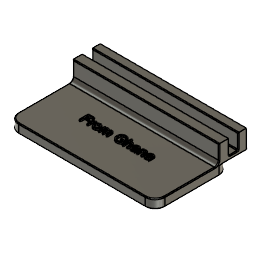
name_tag (Autodesk Fusion 360 design; units mm, degrees)
Autodesk Fusion 360 part; units mm, degrees
sketch "Sketch1" plane through (0, 0, 0) normal (0, 0, 1) x (1, 0, 0)
  line L0 (0, 0) -> (0, 18.796)
  line L1 (0, 0) -> (-86.8649, 0) construction
  line L2 (3.429, 22.225) -> (47.371, 22.225)
  line L3 (25.4, 22.225) -> (25.4, 6.2788) construction
  line L4 (0, 9.398) -> (48.3503, 9.398) construction
  line L5 (3.429, -3.429) -> (47.371, -3.429)
  line L6 (50.8, 0) -> (50.8, 18.796)
  arc A0 (3.429, 22.225) -> (0, 18.796) centre (3.429, 18.796) ccw
  arc A1 (50.8, 18.796) -> (47.371, 22.225) centre (47.371, 18.796) ccw
  arc A2 (47.371, -3.429) -> (50.8, 0) centre (47.371, 0) ccw
  arc A3 (0, 0) -> (3.429, -3.429) centre (3.429, 0) ccw
  dimension "d1" = 18.796
  dimension "d2" = 6.858
  dimension "d3" = 43.942
  constraint coincident L0.start L1.start
  constraint vertical L0
  constraint perpendicular L0 L1
  constraint tangent L0 A0
  constraint horizontal L2
  constraint tangent L2 A0
  constraint midpoint L2 L3.start
  constraint perpendicular L2 L3
  constraint midpoint L0 L4.start
  constraint perpendicular L3 L4
  constraint symmetric L2.start L4 L5.start
  constraint symmetric L2.end L4 L5.end
  constraint symmetric L0.start L3 L6.start
  constraint symmetric L0.end L3 L6.end
  constraint symmetric L3 A0 A1
  constraint symmetric L4 A0 A3
  constraint symmetric L4 A1 A2
  constraint coincident L0 L1.start
  measures "d1" distance of L0.start L0.end
  measures "d2" diameter of A0
  measures "d3" distance of L2.start L2.end
extrude "Extrude1" add sketch "Sketch1" along normal blind 3.175
chamfer "Chamfer1" distance 0.254 angle 45 8 edges at (25.4, -3.429, 0) (49.7957, -2.4247, 0) (50.8, 9.398, 0) (49.7957, 21.2207, 0) (25.4, 22.225, 0) (1.0043, 21.2207, 0) (0, 9.398, 0) (1.0043, -2.4247, 0)
sketch "Sketch2" plane through (0, 0, 3.175) normal (0, 0, 1) x (-1, 0, 0)
  arc A0 (-3.429, -22.225) -> (0, -18.796) centre (-3.429, -18.796) ccw
  line L0 (0, -18.796) -> (0, 0)
  arc A1 (0, 0) -> (-3.429, 3.429) centre (-3.429, 0) ccw
  line L1 (-3.429, 3.429) -> (-47.371, 3.429)
  arc A2 (-47.371, 3.429) -> (-50.8, 0) centre (-47.371, 0) ccw
  line L2 (-50.8, 0) -> (-50.8, -18.796)
  arc A3 (-50.8, -18.796) -> (-47.371, -22.225) centre (-47.371, -18.796) ccw
  line L3 (-47.371, -22.225) -> (-3.429, -22.225)
  line L4 (-3.429, -18.796) -> (-47.371, -18.796)
  line L5 (-3.429, 0) -> (-47.371, 0)
  line L6 (-3.429, 0) -> (-47.371, 0) construction
  line L7 (-47.371, 0) -> (-47.371, -18.796) construction
  line L8 (-47.371, -18.796) -> (-3.429, -18.796) construction
  line L9 (-3.429, -18.796) -> (-3.429, 0) construction
  dimension "d7" = 3.175
  text T0 "From Ghana" font "Arial" height 3.175 align centre middle in box 43.942 x 18.796 at (-3.429, 0) x (-1, 0) y (0, -1) spacing 1 kerned
  constraint coincident A0.centre L4.start
  constraint coincident A3.centre L4.end
  constraint coincident A1.centre L5.start
  constraint coincident A2.centre L5.end
  constraint coincident A2.centre
  constraint coincident A0.centre
sketch "Sketch3" plane through (50.8, 0, 0) normal (1, 0, 0) x (0, 1, 0)
  line L0 (0, 0.254) -> (18.796, 0.254)
  line L1 (18.796, 0.254) -> (18.796, 3.175)
  line L2 (18.796, 3.175) -> (0, 3.175)
  line L3 (0, 3.175) -> (0, 0.254)
  line L4 (18.796, 3.175) -> (28.575, 3.175)
  line L5 (22.225, 0.254) -> (22.225, 3.175)
  line L6 (28.575, 3.175) -> (28.575, 9.5956)
  line L7 (28.575, 9.5956) -> (18.796, 9.5956)
  line L8 (18.796, 9.5956) -> (18.796, 3.175)
  dimension "d9" = 6.35
  constraint coincident L1.end L2.start
  constraint perpendicular L1 L4
  constraint perpendicular L4 L6
  constraint perpendicular L6 L7
  constraint vertical L8
  measures "d9" distance of L4.end L5.end
extrude "Extrude2" add sketch "Sketch3" against normal blind 50.8 contours L4 L6 L7 L8
fillet "Fillet1" radius 1.397 1 edges at (25.4, 18.796, 3.175)
fillet "Fillet1" radius 0.1778 3 edges at (49.7957, 21.2207, 3.175) (25.4, 22.225, 3.175) (1.0043, 21.2207, 3.175)
sketch "Sketch4" plane through (50.8, 0, 0) normal (1, 0, 0) x (0, 1, 0)
  line L0 (0, 0.254) -> (18.796, 0.254)
  line L1 (18.796, 0.254) -> (18.796, 2.9972)
  spline S0 degree 3 poles (19.9145, 3.175) (19.5586, 3.175) (19.143, 3.0762) (18.796, 2.9972) knots 0.210447 0.210447 0.210447 0.210447 0.317222 0.317222 0.317222 0.317222
  line L2 (19.9145, 3.175) -> (28.575, 3.175)
  line L3 (28.575, 3.175) -> (28.575, 9.5956)
  line L4 (28.575, 9.5956) -> (18.796, 9.5956)
  line L5 (18.796, 9.5956) -> (18.796, 4.572)
  arc A0 (17.399, 3.175) -> (18.796, 4.572) centre (17.399, 4.572) ccw
  line L6 (17.399, 3.175) -> (0, 3.175)
  line L7 (0, 3.175) -> (0, 0.254)
  line L8 (22.225, 0.254) -> (22.225, 2.9972)
  line L9 (22.225, 2.9972) -> (22.225, 9.5956)
  line L10 (25.4914, 4.2669) -> (22.291, 4.2669)
  line L11 (22.291, 4.2669) -> (22.291, 9.5956)
  line L12 (22.291, 9.5956) -> (25.4914, 9.5956)
  line L13 (25.4914, 9.5956) -> (25.4914, 4.2669)
  dimension "d22" = 3.2004
  constraint coincident L8.end L9.start
  constraint coincident L4 L9.end
  constraint perpendicular L4 L9
  constraint horizontal L10
  constraint vertical L11
  constraint horizontal L12
  constraint vertical L13
  constraint coincident L9.end L12
  measures "d22" distance of L11 L13
extrude "Extrude3" cut sketch "Sketch4" against normal blind 50.8 contours L4 L10 L11 L12 L13
fillet "Fillet2" radius 0.254 3 faces at (33.8667, 22.291, 6.0431) (33.8667, 24.4246, 4.2669) (33.8667, 25.4914, 7.8193)
fillet "Fillet3" radius 0.254 4 faces at (33.8667, 28.575, 5.3152) (33.8667, 18.796, 7.921) (16.9333, 17.5318, 3.1813) (18.0763, 10.4563, 3.175)
extrude "Extrude4" add sketch "Sketch2" along normal blind 0.508 text T0
equation "d2 = ( 0.135 * 2 ) * 1 in"
equation "d8 = 'From Ghana'"
